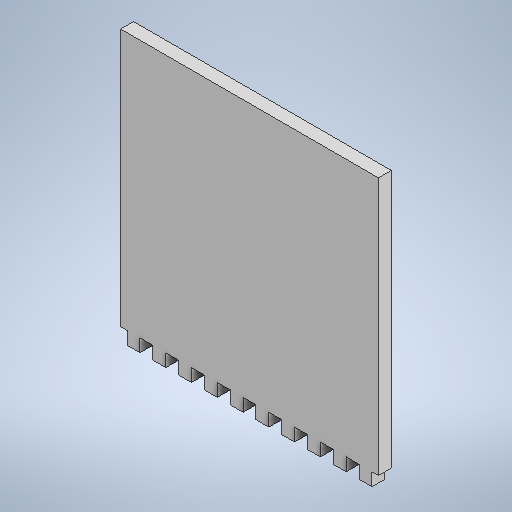
# Autodesk Inventor part: wall inteface V1
Saved by Autodesk Inventor 2025.3 (Build 293356000, 356)
## iProperties
Created: 2026-05-02
Part Number: wall inteface V1
Material: Generic
Document SubType Name: Modeling
Designer: kamal
Density: 1 g/cm^3
Appearance: Default
Author: kamal
Autodesk Inventor part; units mm, degrees
ref_plane "YZ Plane" through (0, 0, 0) normal (1, 0, 0) x (0, 1, 0)
ref_plane "XZ Plane" through (0, 0, 0) normal (0, 1, 0) x (-1, 0, 0)
ref_plane "XY Plane" through (0, 0, 0) normal (0, 0, 1) x (1, 0, 0)
sketch "Sketch1" plane through (0, 0, 0) normal (0, 0, 1) x (1, 0, 0)
  line L0 (0, 6) -> (120, 6)
  line L1 (120, 6) -> (120, 0)
  line L2 (120, 0) -> (0, 0)
  line L3 (0, 0) -> (0, 6)
  line L4 (3, 6) -> (3, 0)
  line L5 (9, 6) -> (9, 0)
  line L6 (9, 6) -> (9, 0)
  line L7 (15, 6) -> (15, 0)
  line L8 (15, 6) -> (15, 0)
  line L9 (21, 6) -> (21, 0)
  line L10 (21, 6) -> (21, 0)
  line L11 (27, 6) -> (27, 0)
  line L12 (27, 6) -> (27, 0)
  line L13 (33, 6) -> (33, 0)
  line L14 (33, 6) -> (33, 0)
  line L15 (39, 6) -> (39, 0)
  line L16 (39, 6) -> (39, 0)
  line L17 (45, 6) -> (45, 0)
  line L18 (45, 6) -> (45, 0)
  line L19 (51, 6) -> (51, 0)
  line L20 (51, 6) -> (51, 0)
  line L21 (57, 6) -> (57, 0)
  line L22 (57, 6) -> (57, 0)
  line L23 (63, 6) -> (63, 0)
  line L24 (63, 6) -> (63, 0)
  line L25 (69, 6) -> (69, 0)
  line L26 (69, 6) -> (69, 0)
  line L27 (75, 6) -> (75, 0)
  line L28 (75, 6) -> (75, 0)
  line L29 (81, 6) -> (81, 0)
  line L30 (81, 6) -> (81, 0)
  line L31 (87, 6) -> (87, 0)
  line L32 (87, 6) -> (87, 0)
  line L33 (93, 6) -> (93, 0)
  line L34 (93, 6) -> (93, 0)
  line L35 (99, 6) -> (99, 0)
  line L36 (99, 6) -> (99, 0)
  line L37 (105, 6) -> (105, 0)
  line L38 (105, 6) -> (105, 0)
  line L39 (111, 6) -> (111, 0)
  line L40 (111, 6) -> (111, 0)
  line L41 (117, 6) -> (117, 0)
  line L42 (0, 6) -> (0, 126)
  line L43 (120, 6) -> (120, 126)
  line L44 (120, 126) -> (0, 126)
  point P0 (0, 3)
  point P1 (3, 3)
  point P2 (9, 3)
  point P3 (15, 3)
  point P4 (21, 3)
  point P5 (27, 3)
  point P6 (33, 3)
  point P7 (39, 3)
  point P8 (45, 3)
  point P9 (51, 3)
  point P10 (57, 3)
  point P11 (63, 3)
  point P12 (69, 3)
  point P13 (75, 3)
  point P14 (81, 3)
  point P15 (87, 3)
  point P16 (93, 3)
  point P17 (99, 3)
  point P18 (105, 3)
  point P19 (111, 3)
  dimension "d4" = 120
  dimension "d5" = 6
  dimension "d6" = 3
  dimension "d7" = 6
  dimension "d8" = 6
  dimension "d10" = 120
  dimension "d11" = 120
  constraints: 90 horizontal alignment, 86 end point, 37 parallel, 5 vertical, 2 midpoint, 1 coincident, 10 other
  measures "d4" distance of L1.end L3.start
  measures "d5" distance of L1.start L1.end
  measures "d6" distance of point (0, 3) point (3, 3)
  measures "d7" distance between parallel lines of L5 L4
  measures "d8" distance of L4.start L6.start
  measures "d10" distance of L3.end L42.end
  measures "d11" distance of L1.start L43.end
extrude "Extrusion1" add sketch "Sketch1" along normal blind 6 contours L42 L44 L43 L0 | L0 L5 L2 L4 | L0 L9 L2 L7 | L41 L2 L39 L0 | L0 L13 L2 L11 | L37 L2 L35 L0 | L0 L17 L2 L15 | L33 L2 L31 L0 | L0 L21 L2 L19 | L29 L2 L27 L0 | L0 L25 L2 L23
body "Solid1"
